BLDCMotor (Autodesk Fusion 360 design; units mm, degrees)
Autodesk Fusion 360 part; units mm, degrees
sketch "Sketch1" plane through (0, 0, 0) normal (0, 0, 1) x (1, 0, 0)
  circle A0 centre (0, 0) radius 13.9
  dimension "d1" = 27.8
  constraint coincident A0.centre origin
  measures "d1" diameter of A0
extrude "Extrude1" add sketch "Sketch1" along normal blind 13
sketch "Sketch2" plane through (0, 0, 13) normal (0, 0, 1) x (-1, 0, 0)
  circle A0 centre (0, 0) radius 13.9
  circle A1 centre (0, 0) radius 1.7
  dimension "d4" = 3.4
  constraint concentric A0 A1
  measures "d4" diameter of A1
extrude "Extrude2" cut sketch "Sketch2" against normal through all contours A1
sketch "Sketch3" plane through (0, 0, 13) normal (0, 0, 1) x (-1, 0, 0)
  circle A0 centre (0, 0) radius 1.7
  circle A1 centre (0, 0) radius 13.9
  line L0 (-4.25, -4.25) -> (4.25, -4.25) construction
  line L1 (4.25, -4.25) -> (4.25, 4.25) construction
  line L2 (4.25, 4.25) -> (-4.25, 4.25) construction
  line L3 (-4.25, 4.25) -> (-4.25, -4.25) construction
  line L4 (-4.25, -4.25) -> (4.25, 4.25) construction
  line L5 (4.25, -4.25) -> (-4.25, 4.25) construction
  circle A2 centre (4.25, -4.25) radius 1
  circle A3 centre (-4.25, -4.25) radius 1
  circle A4 centre (-4.25, 4.25) radius 1
  circle A5 centre (4.25, 4.25) radius 1
  dimension "d6" = 8.5
  dimension "d7" = 8.5
  dimension "d8" = 2
  dimension "d9" = 2
  dimension "d10" = 2
  dimension "d11" = 2
  constraint horizontal L0
  constraint perpendicular L0 L1
  constraint parallel L0 L2
  constraint parallel L1 L3
  constraint coincident L4 A0.centre
  constraint coincident L5 A0.centre
  constraint coincident A0.centre A1.centre
  constraint coincident L0.end L1.start
  constraint coincident L0.start L3.end
  constraint coincident L2.end L3.start
  constraint coincident L1.end L2.start
  measures "d6" distance of L1.end L2.end
  measures "d7" distance of L0.end L1.end
  measures "d8" diameter of A2
  measures "d9" diameter of A5
  measures "d10" diameter of A3
  measures "d11" diameter of A4
extrude "Extrude3" cut sketch "Sketch3" against normal through all contours A2 | A3 | A4 | A5
sketch "Sketch4" plane through (0, 0, 0) normal (0, 0, -1) x (1, 0, 0)
  circle A0 centre (4.25, -4.25) radius 1
  circle A1 centre (-4.25, 4.25) radius 1
  circle A2 centre (-4.25, -4.25) radius 1
  circle A3 centre (4.25, 4.25) radius 1
  circle A4 centre (0, 0) radius 1.7
  circle A5 centre (0, 0) radius 13.9
  line L0 (0, 0) -> (0, 7.9) construction
  line L1 (-6, 13.9) -> (6, 13.9)
  line L2 (6, 13.9) -> (6, 7.9)
  line L3 (6, 7.9) -> (-6, 7.9)
  line L4 (-6, 7.9) -> (-6, 13.9)
  dimension "d13" = 12
  dimension "d14" = 6
  constraint coincident A4.centre A5.centre
  constraint vertical L0
  constraint horizontal L1
  constraint vertical L2
  constraint horizontal L3
  constraint vertical L4
  constraint midpoint L0.end L3
  constraint tangent A5 L1
  measures "d13" distance of L2.end L3.end
  measures "d14" distance of L1 L3
extrude "Extrude4" cut sketch "Sketch4" against normal blind 2.5 contours A5 L2 L3 L4 picked at (0, 9.9)
sketch "Sketch5" plane through (0, 0, 2.5) normal (0, 0, -1) x (1, 0, 0)
  arc A0 (6, 12.5383) -> (-6, 12.5383) centre (0, 0) ccw
  line L0 (-6, 12.5383) -> (-6, 7.9)
  line L1 (-6, 7.9) -> (6, 7.9)
  line L2 (6, 7.9) -> (6, 12.5383)
  line L3 (-0.75, 12.9) -> (0.75, 12.9)
  line L4 (0.75, 12.9) -> (0.75, 8.9)
  line L5 (0.75, 8.9) -> (-0.75, 8.9)
  line L6 (-0.75, 8.9) -> (-0.75, 12.9)
  line L7 (0, 7.9) -> (0, 8.9) construction
  line L8 (-3.75, 12.9) -> (-2.25, 12.9)
  line L9 (-3.75, 8.9) -> (-3.75, 12.9)
  line L10 (-2.25, 12.9) -> (-2.25, 8.9)
  line L11 (-2.25, 8.9) -> (-3.75, 8.9)
  line L12 (2.25, 12.9) -> (3.75, 12.9)
  line L13 (2.25, 8.9) -> (2.25, 12.9)
  line L14 (3.75, 12.9) -> (3.75, 8.9)
  line L15 (3.75, 8.9) -> (2.25, 8.9)
  dimension "d17" = 1.5
  dimension "d18" = 4
  dimension "d19" = 1
  dimension "d22" = 3
  dimension "d23" = 0
  constraint horizontal L3
  constraint vertical L4
  constraint horizontal L5
  constraint vertical L6
  constraint midpoint L1 L7.start
  constraint midpoint L5 L7.end
  constraint perpendicular L5 L7
  measures "d17" distance of L4.end L5.end
  measures "d18" distance of L3.end L4.end
  measures "d19" distance of L7.start L7.end
extrude "Extrude5" add sketch "Sketch5" along normal blind 0.5 contours L3 L4 L5 L6 | L8 L9 L10 L11 | L12 L13 L14 L15
ref_plane "WorkPlane1" through (0, 0.6808, 4) normal (0, 0, -1) x (-1, 0, 0)
sketch "Sketch6" plane through (0, 0.6808, 4) normal (0, 0, -1) x (1, 0, 0)
  circle A0 centre (0, 0.6808) radius 12.5
  arc A1 (-6, 13.2192) -> (6, 13.2192) centre (0, 0.6808) ccw
  circle A2 centre (0, 0.6808) radius 13.9
  dimension "d27" = 25
  constraint concentric A0 A1
  constraint concentric A0 A2
  constraint coincident A1.end A2
  measures "d27" diameter of A0
extrude "Extrude6" cut sketch "Sketch6" along normal blind 0.5
fillet "Fillet1" radius 0.3 2 edges at (-12.9594, 5.0265, 3.5) (-12.9594, -5.0265, 4)
sketch "Sketch7" plane through (0, 0, 0) normal (0, 0, -1) x (1, 0, 0)
  line L0 (-6, 7.9) -> (-6, 12.5383)
  arc A0 (-6, 12.5383) -> (6, 12.5383) centre (0, 0) ccw
  line L1 (6, 12.5383) -> (6, 7.9)
  line L2 (6, 7.9) -> (-6, 7.9)
  circle A1 centre (4.25, -4.25) radius 1
  circle A2 centre (-4.25, 4.25) radius 1
  circle A3 centre (-4.25, -4.25) radius 1
  circle A4 centre (4.25, 4.25) radius 1
  circle A5 centre (0, 0) radius 1.7
  circle A6 centre (0, 0) radius 4.5
  dimension "d32" = 9
  constraint coincident A0.centre A5.centre
  measures "d32" diameter of A6
extrude "Extrude7" cut sketch "Sketch7" against normal blind 0.5 contours A6
sketch "Sketch8" plane through (0, 0, 13) normal (0, 0, 1) x (-1, 0, 0)
  circle A0 centre (-4.25, -4.25) radius 1
  circle A1 centre (4.25, 4.25) radius 1
  circle A2 centre (4.25, -4.25) radius 1
  circle A3 centre (-4.25, 4.25) radius 1
  circle A4 centre (0, 0) radius 1.7
  circle A5 centre (0, 0) radius 13.9
  circle A6 centre (0, 0) radius 2.25
  circle A7 centre (0, 0) radius 2.3
  dimension "d35" = 4.5
  dimension "d36" = 4.6
  constraint coincident A4.centre A5.centre
  measures "d35" diameter of A6
  measures "d36" diameter of A7
extrude "Extrude8" cut sketch "Sketch8" against normal blind 0.2 contours A7
extrude "Extrude9" cut 1 faces at (-2.052, 0.1962, 13) along direction (0, 0, -1) blind 0.1
move_body "Move1" bodies 1 to x (0, 0, 1) y (0, 1, 0) z (-1, 0, 0) at (12.9, 0, 12.9)
move_body "Move2" bodies 1 to x (-1, 0, 0) y (0, -1, 0) z (0, 0, 1) at (25.8, -8.9178, 0)
move_body "Move3" bodies 1 to x (0, 0, 1) y (0, 1, 0) z (-1, 0, 0) at (38.8, 0, -13)
move_body "Move4" bodies 1 to x (1, 0, 0) y (0, 1, 0) z (0, 0, 1) at (0, 0, 5)
equation "d9 = d8"
equation "d10 = d8"
equation "d11 = d8"
